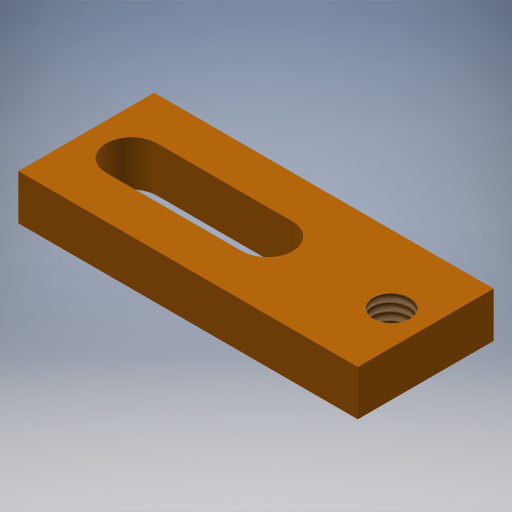
# Autodesk Inventor part: 24_0497_0021
Saved by Autodesk Inventor 2024.3 (Build 283343000, 343)
## iProperties
Created: 2024-07-08
Part Number: 24_0497_0021
Material: Allgemein
Document SubType Name: Modeling
Designer: Vogel
Density: 1 g/cm^3
Appearance: Orange
Author: Vogel
Autodesk Inventor part; units mm, degrees
ref_plane "YZ Plane" through (0, 0, 0) normal (1, 0, 0) x (0, 1, 0)
ref_plane "XZ Plane" through (0, 0, 0) normal (0, 1, 0) x (-1, 0, 0)
ref_plane "XY Plane" through (0, 0, 0) normal (0, 0, 1) x (1, 0, 0)
sketch "Skizze1" plane through (0, 0, 0) normal (0, 0, 1) x (1, 0, 0)
  line L0 (-21, 0) -> (21, 0) projected
  line L1 (0, -8.4) -> (0, 8.4) projected
  line L2 (15, -6) -> (-15, -6)
  line L3 (-15, -6) -> (-15, 6)
  line L4 (-15, 6) -> (15, 6)
  line L5 (15, 6) -> (15, -6)
  line L6 (15, -6) -> (-15, 6) construction
  line L7 (-15, -6) -> (15, 6) construction
  point P0 (0, 0)
  dimension "d0" = 12
  dimension "d1" = 30
  constraints: 12 end point, 2 midpoint, 2 parallel, 1 horizontal, 1 perpendicular
  measures "d0" distance of L2.end L3.end
  measures "d1" distance of L3.end L4.end
extrude "Extrusion1" add sketch "Skizze1" along normal blind 4
sketch "Skizze2" plane through (0, 0, 0) normal (0, 0, -1) x (-1, 0, 0)
  line L0 (15, -6) -> (-15, -6) projected
  line L1 (15, 6) -> (15, -6) projected
  line L2 (-15, 6) -> (15, 6) projected
  line L3 (21, 0) -> (-21, 0) projected
  line L4 (0, -8.4) -> (0, 8.4) projected
  point P0 (0, 0)
  point P1 (-1, 0)
  point P2 (11, 0)
  point P3 (15, 0)
  dimension "d5" = 4
  dimension "d6" = 16
  constraints: 2 point on line, 1 midpoint
  measures "d5" distance of point (11, 0) point (15, 0)
  measures "d6" distance from line of point (-1, 0) L1
hole "Bohrung1" at (1, 0, 0) at (-11, 0, 0) direction (0, 0, 1) diameter 4.5 end through all
sketch "Skizze3" plane through (0, 0, 4) normal (0, 0, 1) x (1, 0, 0)
  circle A0 centre (-11, 0) radius 2.25 projected
  circle A1 centre (1, 0) radius 2.25 projected
  line L0 (-15, -6) -> (15, -6) projected
  line L1 (15, -6) -> (15, 6) projected
  line L2 (15, 6) -> (-15, 6) projected
  line L3 (-15, 6) -> (-15, -6) projected
  line L4 (-21, 0) -> (21, 0) projected
  line L5 (0, -8.4) -> (0, 8.4) projected
  point P0 (0, 0)
  point P1 (12, 0)
  dimension "d14" = 3
  constraints: 1 point on line
  measures "d14" distance from line of point (12, 0) L1
hole "Bohrung2" at (12, 0, 4) direction (0, 0, -1) diameter 3.242 end through all thread size "M4x0.7" class "6H" standard "ISO Metric profile"
sketch "Skizze4" plane through (0, 0, 4) normal (0, 0, 1) x (1, 0, 0)
  circle A0 centre (12, 0) radius 1.621 projected
  circle A1 centre (-11, 0) radius 2.25 projected
  circle A2 centre (1, 0) radius 2.25 projected
  line L0 (-15, -6) -> (15, -6) projected
  line L1 (15, -6) -> (15, 6) projected
  line L2 (15, 6) -> (-15, 6) projected
  line L3 (-15, 6) -> (-15, -6) projected
  line L4 (-11, 2.25) -> (1, 2.25)
  line L5 (1, 2.25) -> (1, -2.25)
  line L6 (1, -2.25) -> (-11, -2.25)
  line L7 (-11, -2.25) -> (-11, 2.25)
  circle A3 centre (1, 0) radius 2.25 projected
  point P0 (0, 0)
  constraints: 8 end point, 2 horizontal, 2 parallel, 1 perpendicular, 1 tangent, 4 other
extrude "Extrusion2" cut sketch "Skizze4" against normal through all contours A1 L4 A2 L6
